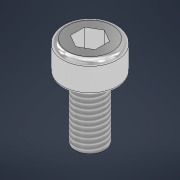
# Autodesk Inventor part: M3-CapScrew
Saved by Autodesk Inventor 2022.5 (Build 265521000, 521)
## iProperties
Created: 2022-02-28
Part Number: M3-CapScrew
Material: 一般
Document SubType Name: Modeling
Designer: Yuta Fujiyama
Density: 7.18875 g/cm^3
Appearance: クローム - つや出し
Mass: 0.732 g
Surface Area: 1.67902 cm^2
Volume: 0.101826 cm^3
Author: Yuta Fujiyama
Autodesk Inventor part; units mm, degrees
ref_plane "YZ Plane" through (0, 0, 0) normal (1, 0, 0) x (0, 1, 0)
ref_plane "XZ Plane" through (0, 0, 0) normal (0, 1, 0) x (-1, 0, 0)
ref_plane "XY Plane" through (0, 0, 0) normal (0, 0, 1) x (1, 0, 0)
sketch "スケッチ1" plane through (0, 0, 0) normal (0, 1, 0) x (-1, 0, 0)
  circle A0 centre (0, 0) radius 2.75
  dimension "d0" = 5.5
  constraints: 1 centre point, 1 coincident
  measures "d0" diameter of A0
extrude "押し出し1" add sketch "スケッチ1" along normal blind 3
sketch "スケッチ2" plane through (0, 0, 0) normal (0, -1, 0) x (1, 0, 0)
  circle A0 centre (0, 0) radius 1.5
  dimension "d3" = 3
  constraints: 1 centre point, 1 coincident
  measures "d3" diameter of A0
extrude "押し出し2" add sketch "スケッチ2" along normal blind 6
fillet "フィレット1" radius 0.5 1 edges at (2.75, 3, 0)
fillet "フィレット1" radius 0.2 1 edges at (2.75, 0, 0)
sketch "スケッチ3" plane through (0, 3, 0) normal (0, 1, 0) x (1, 0, 0)
  line L0 (0, 1.4434) -> (-1.25, 0.7217)
  line L1 (-1.25, 0.7217) -> (-1.25, -0.7217)
  line L2 (-1.25, -0.7217) -> (0, -1.4434)
  line L3 (0, -1.4434) -> (1.25, -0.7217)
  line L4 (1.25, -0.7217) -> (1.25, 0.7217)
  line L5 (1.25, 0.7217) -> (0, 1.4434)
  line L6 (0, 1.4434) -> (0, -1.4434) construction
  circle A0 centre (0, 0) radius 1.4434 construction
  dimension "d12" = 2.5
  constraints: 14 end point, 5 point on circle, 3 equal length, 2 coincident, 1 centre point, 1 midpoint, 1 parallel, 1 vertical
  measures "d12" distance between parallel lines of L4 L1
extrude "押し出し3" cut sketch "スケッチ3" against normal blind 2
thread "ねじ1" size "M3x0.5" class "6g" standard "ANSI Metric M Profile" full length
